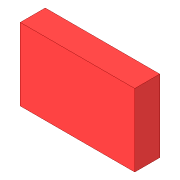
# Autodesk Inventor part: ‎BOB-15100‎ USB C Breakout
Saved by Autodesk Inventor 2018.3 (Build 223284000, 284)
## iProperties
Created: 2018-12-11
Part Number: ‎BOB-15100‎ USB C Breakout
Material: Generic
Document SubType Name: Modeling
Designer: tei06398
Mass: 1.48983 g
Surface Area: 9.65546 cm^2
Volume: 1.48983 cm^3
Density: 1 g/cm^3
Appearance: Default
Author: tei06398
Autodesk Inventor part; units mm, degrees
ref_plane "YZ Plane" through (0, 0, 0) normal (1, 0, 0) x (0, 1, 0)
ref_plane "XZ Plane" through (0, 0, 0) normal (0, 1, 0) x (-1, 0, 0)
ref_plane "XY Plane" through (0, 0, 0) normal (0, 0, 1) x (1, 0, 0)
sketch "Sketch1" plane through (0, 0, 0) normal (0, 0, 1) x (1, 0, 0)
  line L0 (0, 0) -> (22.098, 0)
  line L1 (22.098, 0) -> (22.098, 13.97)
  line L2 (22.098, 13.97) -> (0, 13.97)
  line L3 (0, 13.97) -> (0, 0)
  dimension "d0" = 22.098
  dimension "d1" = 13.97
  constraints: 8 end point, 2 parallel, 1 horizontal, 1 perpendicular
  measures "d0" distance of L2.end L1.end
  measures "d1" distance of L1.end L0.end
extrude "Extrusion1" add sketch "Sketch1" against normal blind 4.826
body "Solid1"
